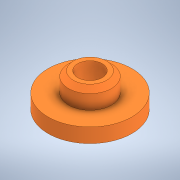
# Autodesk Inventor part: Indre_bøsning_Stempel_stang
Saved by Autodesk Inventor 2022 (Build 260153000, 153)
## iProperties
Created: 2022-05-04
Part Number: Indre_bøsning_Stempel_stang
Material: Generic
Document SubType Name: Modeling
Designer: Patrick
Density: 1 g/cm^3
Appearance: Default
Author: Patrick
Autodesk Inventor part; units mm, degrees
ref_plane "YZ Plane" through (0, 0, 0) normal (1, 0, 0) x (0, 1, 0)
ref_plane "XZ Plane" through (0, 0, 0) normal (0, 1, 0) x (-1, 0, 0)
ref_plane "XY Plane" through (0, 0, 0) normal (0, 0, 1) x (1, 0, 0)
sketch "Sketch1" plane through (0, 0, 0) normal (0, 1, 0) x (-1, 0, 0)
  circle A0 centre (0, 0) radius 5.1
  circle A1 centre (0, 0) radius 8.95
  dimension "d0" = 10.2
  dimension "d1" = 17.9
  constraints: 2 centre point, 2 coincident
  measures "d0" diameter of A0
  measures "d1" diameter of A1
extrude "Extrusion1" add sketch "Sketch1" along normal blind 8
chamfer "Chamfer1" distance 2 angle 45 1 edges at (8.95, 8, 0)
sketch "Sketch2" plane through (0, 0, 0) normal (0, -1, 0) x (1, 0, 0)
  circle A0 centre (0, 0) radius 8.95 projected
  circle A1 centre (0, 0) radius 5.1 projected
  circle A2 centre (0, 0) radius 17.5
  dimension "d7" = 35
  constraints: 1 centre point, 1 coincident
  measures "d7" diameter of A2
extrude "Extrusion2" add sketch "Sketch2" along normal blind 6 contours A0 | A2
body "Solid1"
